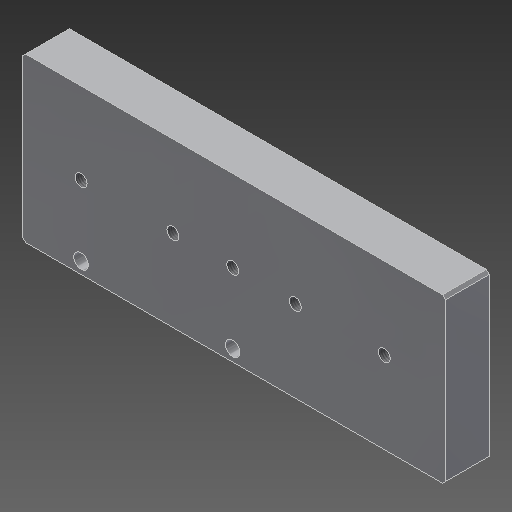
# Autodesk Inventor part: 02
Saved by Autodesk Inventor 2021.1 (Build 251245010, 245A)
## iProperties
Created: 2008-11-14
Part Number: 02
Document SubType Name: Modeling
Density: 2.71 g/cm^3
Material: A5052
Mass: 879.09 g
Surface Area: 549.129 cm^2
Volume: 324.387 cm^3
Appearance: アルミニウム - フラット
個数: 1
尺度: 1:2
Title: プレート
Autodesk Inventor part; units mm, degrees
ref_plane "YZ Plane" through (0, 0, 0) normal (1, 0, 0) x (0, 1, 0)
ref_plane "XZ Plane" through (0, 0, 0) normal (0, 1, 0) x (-1, 0, 0)
ref_plane "XY Plane" through (0, 0, 0) normal (0, 0, 1) x (1, 0, 0)
sketch "スケッチ1" plane through (0, 0, 0) normal (0, 0, 1) x (1, 0, 0)
  line L0 (-72.5, -28) -> (72.5, -28)
  line L1 (72.5, -28) -> (72.5, 28)
  line L2 (72.5, 28) -> (-72.5, 28)
  line L3 (-72.5, 28) -> (-72.5, -28)
  point P0 (0, 0)
  point P1 (0, -28)
  point P2 (-72.5, 0)
  dimension "d0" = 145
  dimension "d1" = 56
  constraints: 8 end point, 2 midpoint, 2 parallel, 1 horizontal, 1 horizontal alignment, 1 perpendicular, 1 vertical alignment
  measures "d0" distance of L0.start L0.end
  measures "d1" distance of L2.end L0.start
extrude "押し出し1" add sketch "スケッチ1" along normal blind 15
sketch "スケッチ3" plane through (0, 0, 15) normal (0, 0, 1) x (1, 0, 0)
  point P0 (0, 0)
  point P1 (-21, 0)
  point P2 (21, 0)
  dimension "d9" = 21
  dimension "d10" = 21
  constraints: 2 horizontal alignment
  measures "d9" distance of point (0, 0) point (-21, 0)
  measures "d10" distance of point (21, 0) point (0, 0)
hole "穴1" at (-21, 0, 15) at (21, 0, 15) direction (0, 0, -1) diameter 4.134 end through all thread size "M5x0.8" class "6H" standard "ANSI Metric M Profile"
sketch "スケッチ4" plane through (0, 0, 0) normal (0, 0, -1) x (-1, 0, 0)
  line L0 (-72.5, -28) -> (-72.5, 28) projected
  point P0 (0, 0)
  point P1 (-51.5, 0)
  point P2 (-72.5, 0)
  dimension "d18" = 21
  constraints: 1 horizontal alignment, 1 midpoint
  measures "d18" distance from line of point (-51.5, 0) L0
hole "穴2" at (51.5, 0, 0) direction (0, 0, 1) diameter 4.134 end through all thread size "M5x0.8" class "6H" standard "ANSI Metric M Profile"
pattern_linear "矩形状パターン1" count 3 spacing 52 along (-1, 0, 0) of "穴2"
sketch "スケッチ5" plane through (0, 0, 0) normal (0, 0, -1) x (-1, 0, 0)
  circle A0 centre (52.5, 0) radius 2.067 projected
  circle A1 centre (0.5, 0) radius 2.067 projected
  point P0 (0, 0)
  point P1 (52.5, -24)
  point P2 (0.5, -24)
  dimension "d29" = 24
  constraints: 2 vertical alignment, 1 horizontal alignment
  measures "d29" distance of point (52.5, -24) A0.centre
hole "穴3" at (-52.5, -24, 0) at (-0.5, -24, 0) direction (0, 0, 1) diameter 5 end through all
chamfer "面取り1" distance 1 angle 45 4 edges at (-72.5, -28, 7.5) (-72.5, 28, 7.5) (72.5, -28, 7.5) (72.5, 28, 7.5)
equation "\"d10\" = d9"
